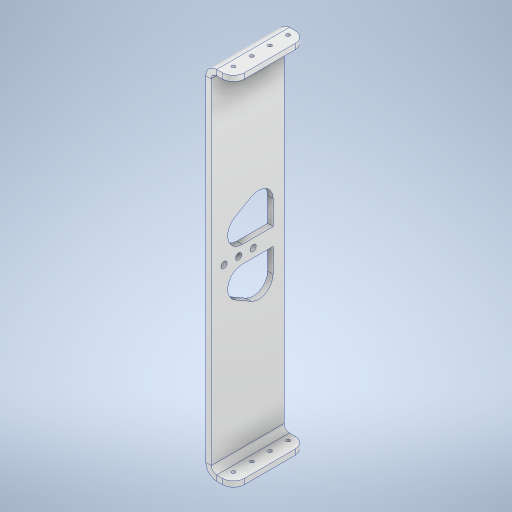
# Autodesk Inventor part: ramp
Saved by Autodesk Inventor 2023 (Build 270158000, 158)
## iProperties
Created: 2022-05-09
Part Number: ramp
Material: Aluminum 6061
Document SubType Name: Sheet Metal
Designer: Dan
Density: 2.7 g/cm^3
Sheet Metal Rule: Default_mm
Appearance: Aluminum - Flat
Mass: 207.914 g
Surface Area: 535.297 cm^2
Volume: 77.0053 cm^3
BendRadius: 3.000 mm
BendReliefWidth: 3.000 mm
BendReliefDepth: 1.500 mm
CornerReliefSize: 12.000 mm
MinimumRemnant: 6.000 mm
TransitionRadius: 3.000 mm
JacobiRadiusSize: 3.000 mm
GapSize: 3.000 mm
Author: Dan
Autodesk Inventor part; units mm, degrees
ref_plane "YZ Plane" through (0, 0, 0) normal (1, 0, 0) x (0, 1, 0)
ref_plane "XZ Plane" through (0, 0, 0) normal (0, 1, 0) x (-1, 0, 0)
ref_plane "XY Plane" through (0, 0, 0) normal (0, 0, 1) x (1, 0, 0)
sketch "Sketch1" plane through (0, 0, 0) normal (0, 1, 0) x (-1, 0, 0)
  line L0 (0, 0) -> (-108, 0)
  line L1 (-108, -40) -> (0, -40)
  line L2 (0, 0) -> (0, -40)
  circle A0 centre (-102, -36) radius 1
  line L3 (-92, -40) -> (-92, 0)
  line L4 (-102, -40) -> (-102, 0) construction
  circle A1 centre (-102, -26) radius 1
  circle A2 centre (-102, -16) radius 1
  circle A3 centre (-102, -6) radius 1
  line L5 (-102, -36) -> (-102, -26)
  line L6 (-92, -40) -> (0, -40)
  line L7 (0, -40) -> (0, -50)
  line L8 (0, -50) -> (-92, -50)
  line L9 (-92, -50) -> (-92, -40)
  line L10 (-108, -40) -> (-108, 0)
  dimension "d50" = 2
  dimension "d84" = 10
  dimension "d87" = 10
  dimension "d92" = 6
  dimension "d96" = 92
  dimension "d97" = 40
  dimension "d132" = 10
  dimension "d151" = 6
  dimension "d152" = 90
  constraints: 23 end point, 5 parallel, 4 centre point, 4 point on line, 2 coincident, 2 horizontal, 2 vertical, 1 perpendicular, 6 other
  measures "d50" diameter of A0
  measures "d84" distance between parallel lines of L3 L4
  measures "d87" distance of L5.start L5.end
  measures "d92" distance from line of L0 A3.centre
  measures "d96" distance of L3.start L1.end
  measures "d97" distance of L0.start L1.end
  measures "d132" distance of L3.start L8.end
  measures "d151" distance between parallel lines of L10 L4
  measures "d152" angle of L6 L3
extrude "Plate1" add sketch "Sketch1" along normal blind 3 contours L2 L1 L3 L0 | L3 L1 L10 L0
fold "Fold2" angle 90 bend radius 3 thickness 3 k factor 0.44 line from (92, 0, -40) to (92, 0, 0) line at bend end moving side (-1, 0, 0) folds toward (0, -1, 0)
fillet "Corner Round2" radius 6 2 edges at (108, 1.5, -40) (108, 1.5, 0)
mirror "Mirror2" about plane through (95.7858, -95, 0) normal (0, -1, 0)
sketch "Sketch17" plane through (92.7858, -187, -40) normal (-1, 0, 0) x (0, 0, 1)
  line L0 (0, 184) -> (0, 0) projected
  line L1 (0, 92) -> (50, 92) construction
  line L2 (0, 190) -> (40, 190) projected
  line L3 (6, -6) -> (34, -6) projected
  line L4 (40, 0) -> (40, 184) projected
  point P0 (40, 187)
  point P1 (17, 92)
  point P2 (25, 92)
  point P3 (33, 92)
  point P4 (25, 92)
  dimension "d174" = 8
  dimension "d175" = 8
  dimension "d178" = 15
  constraints: 2 end point, 2 midpoint, 2 point on line, 1 coincident, 1 horizontal
  measures "d174" distance of point (17, 92) point (25, 92)
  measures "d175" distance of point (33, 92) point (25, 92)
  measures "d178" distance from line of L4 point (25, 92)
hole "Hole2" at (92.7858, -95, -23) at (92.7858, -95, -15) at (92.7858, -95, -7) direction (1, 0, 0) diameter 3.4 end through all clearance for "Countersunk Flat Head Screw ISO 2009/7046" size "M3" standard "ISO"
sketch "Sketch16" plane through (92.7858, -187, -40) normal (-1, 0, 0) x (0, 0, 1)
  line L0 (0, 184) -> (0, 0) projected
  line L1 (0, 92) -> (40, 92) construction
  line L2 (40, 184) -> (40, 0) projected
  line L3 (6, 190) -> (34, 190) projected
  line L4 (20, 190) -> (20, -18.1714) construction
  point P0 (40, 187)
  point P1 (20, 104.75)
  point P2 (20, 79.25)
  dimension "d164" = 25.5
  constraints: 4 end point, 3 midpoint, 1 point on line, 1 symmetric about line, 1 vertical
  measures "d164" distance of point (20, 79.25) point (20, 104.75)
hole "Hole1" [suppressed]
sketch "Sketch18" plane through (92.7858, -187, -40) normal (-1, 0, 0) x (0, 0, 1)
  line L0 (40, 184) -> (40, 0) projected
  line L1 (40, 92) -> (0, 92) construction
  line L2 (0, 184) -> (0, 0) projected
  arc A0 (23, 96.75) -> (27, 111.6782) centre (23, 104.75) ccw
  line L3 (23, 96.75) -> (6, 96.75)
  line L4 (6, 96.75) -> (6, 109.9462)
  arc A1 (18, 116.8744) -> (6, 109.9462) centre (14, 109.9462) ccw
  line L5 (18, 116.8744) -> (27, 111.6782)
  line L6 (40, 0) -> (0, 0) projected
  line L7 (20, 0) -> (20, 184) construction
  line L8 (40, 184) -> (0, 184) projected
  arc A2 (27, 72.3218) -> (23, 87.25) centre (23, 79.25) ccw
  line L9 (23, 87.25) -> (6, 87.25)
  line L10 (6, 87.25) -> (6, 74.0538)
  arc A3 (6, 74.0538) -> (18, 67.1256) centre (14, 74.0538) ccw
  line L11 (18, 67.1256) -> (27, 72.3218)
  point P0 (40, 187)
  dimension "d179" = 16
  dimension "d180" = 12.75
  dimension "d185" = 8
  dimension "d186" = 6
  dimension "d187" = 60
  dimension "d188" = 3
  constraints: 16 end point, 10 point on circle, 8 symmetric about line, 4 centre point, 4 midpoint, 4 tangent, 2 point on line, 1 horizontal, 1 perpendicular, 2 other
  measures "d179" diameter of A0
  measures "d180" distance from line of L1 A0.centre
  measures "d185" radius of A1
  measures "d186" distance between parallel lines of L2 L4
  measures "d187" angle of L7 L5
  measures "d188" distance from line of L7 A0.centre
extrude "Cut5" cut sketch "Sketch18" against normal blind 3 contours L3 L4 A1 L5 A0
extrude "Cut6" cut sketch "Sketch18" against normal blind 3 contours L11 A3 L10 L9 A2
equation "\"d2\" = Thickness"
equation "\"d98\" = BendReliefWidth"
equation "\"d99\" = BendReliefDepth"
equation "\"d100\" = MinimumRemnant"
equation "\"d101\" = TransitionRadius"
equation "\"d103\" = BendRadius"
equation "\"BendRadius\" = Thickness"
equation "\"BendReliefWidth\" = Thickness"
equation "\"BendReliefDepth\" = 0.5 * Thickness"
equation "\"CornerReliefSize\" = 4 * Thickness"
equation "\"MinimumRemnant\" = 2 * Thickness"
equation "\"TransitionRadius\" = BendRadius"
equation "\"JacobiRadiusSize\" = BendRadius"
equation "\"GapSize\" = Thickness"
equation "\"Thickness\" = 3"
body "Solid1"
